Autodesk Fusion 360 part; units mm, degrees
note: some values were not read from the file. Set by a fixed rule: which sketch regions a step uses.
(part 2 of 2)
  spline S9 degree 5 poles (41.1532, -1.6486) (41.1603, -1.6542) (41.1746, -1.6654) (41.1961, -1.6821) (41.2247, -1.7041) (41.2607, -1.7314) (41.2967, -1.7583) (41.3329, -1.7849) (41.3691, -1.8112) (41.4054, -1.8372) (41.4419, -1.8628) (41.4784, -1.8881) (41.515, -1.9131) (41.5517, -1.9378) (41.5885, -1.9621) (41.6254, -1.9861) (41.6623, -2.0097) (41.6994, -2.033) (41.7365, -2.056) (41.7737, -2.0786) (41.811, -2.1009) (41.8483, -2.1229) (41.8857, -2.1445) (41.9232, -2.1657) (41.9608, -2.1866) (41.9984, -2.2071) (42.0361, -2.2273) (42.0738, -2.2471) (42.1116, -2.2666) (42.1495, -2.2857) (42.1874, -2.3044) (42.2254, -2.3227) (42.2634, -2.3407) (42.3014, -2.3583) (42.3395, -2.3755) (42.3777, -2.3923) (42.4158, -2.4088) (42.4541, -2.4248) (42.4923, -2.4405) (42.5306, -2.4558) (42.5689, -2.4706) (42.6072, -2.4851) (42.6456, -2.4991) (42.684, -2.5127) (42.7224, -2.5259) (42.7608, -2.5387) (42.7992, -2.551) (42.8377, -2.563) (42.8761, -2.5745) (42.9145, -2.5855) (42.953, -2.5961) (42.9914, -2.6063) (43.0299, -2.6159) (43.0683, -2.625) (43.1067, -2.6336) (43.145, -2.6417) (43.1834, -2.6494) (43.2217, -2.6566) (43.2601, -2.6634) (43.2983, -2.6697) (43.3366, -2.6753) (43.3747, -2.6802) (43.4128, -2.6844) (43.4508, -2.6877) (43.4888, -2.6904) (43.5266, -2.6925) (43.5644, -2.6943) (43.6022, -2.6956) (43.6398, -2.6965) (43.6773, -2.6964) (43.7146, -2.6948) (43.7442, -2.6918) (43.7662, -2.6883) (43.7808, -2.6855) (43.7881, -2.684) knots -1 -1 -1 -1 -1 -1 -0.98571429 -0.97142857 -0.95714286 -0.94285714 -0.92857143 -0.91428571 -0.9 -0.88571429 -0.87142857 -0.85714286 -0.84285714 -0.82857143 -0.81428571 -0.8 -0.78571429 -0.77142857 -0.75714286 -0.74285714 -0.72857143 -0.71428571 -0.7 -0.68571429 -0.67142857 -0.65714286 -0.64285714 -0.62857143 -0.61428571 -0.6 -0.58571429 -0.57142857 -0.55714286 -0.54285714 -0.52857143 -0.51428571 -0.5 -0.48571429 -0.47142857 -0.45714286 -0.44285714 -0.42857143 -0.41428571 -0.4 -0.38571429 -0.37142857 -0.35714286 -0.34285714 -0.32857143 -0.31428571 -0.3 -0.28571429 -0.27142857 -0.25714286 -0.24285714 -0.22857143 -0.21428571 -0.2 -0.18571429 -0.17142857 -0.15714286 -0.14285714 -0.12857143 -0.11428571 -0.1 -0.08571429 -0.07142857 -0.05714286 -0.04285714 -0.02857143 -0.01428571 0 0 0 0 0 0
  line L9 (43.7881, -2.684) -> (44.8114, -2.4656)
  arc A19 (45.9543, -3.0869) -> (44.8114, -2.4656) centre (45.0201, -3.4436) ccw
  arc A20 (45.9543, -3.0869) -> (46.0732, -3.3739) centre (51.1385, -1.1076) ccw
  arc A21 (45.7044, -4.6213) -> (46.0732, -3.3739) centre (45.1604, -3.7822) ccw
  line L10 (45.7044, -4.6213) -> (44.8264, -5.1905)
  spline S10 degree 5 poles (44.8264, -5.1905) (44.8201, -5.1946) (44.8078, -5.2029) (44.7898, -5.2161) (44.7668, -5.2349) (44.7393, -5.2601) (44.7127, -5.2865) (44.6866, -5.3138) (44.6609, -5.3414) (44.6354, -5.3694) (44.6102, -5.3977) (44.5852, -5.4264) (44.5607, -5.4557) (44.5367, -5.4855) (44.5132, -5.516) (44.4902, -5.547) (44.4675, -5.5785) (44.4452, -5.6104) (44.4232, -5.6426) (44.4015, -5.6751) (44.3801, -5.708) (44.3591, -5.7413) (44.3384, -5.7749) (44.318, -5.8088) (44.298, -5.8432) (44.2783, -5.8778) (44.2589, -5.9129) (44.2399, -5.9482) (44.2211, -5.9838) (44.2027, -6.0197) (44.1845, -6.0559) (44.1667, -6.0924) (44.1492, -6.1291) (44.132, -6.1662) (44.1151, -6.2035) (44.0985, -6.2411) (44.0823, -6.279) (44.0663, -6.3171) (44.0506, -6.3555) (44.0353, -6.3941) (44.0202, -6.433) (44.0054, -6.4721) (43.9909, -6.5114) (43.9768, -6.551) (43.9629, -6.5908) (43.9493, -6.6309) (43.9361, -6.6711) (43.9231, -6.7116) (43.9104, -6.7523) (43.898, -6.7932) (43.886, -6.8344) (43.8742, -6.8757) (43.8627, -6.9172) (43.8515, -6.9589) (43.8406, -7.0009) (43.83, -7.043) (43.8197, -7.0853) (43.8097, -7.1278) (43.8, -7.1705) (43.7906, -7.2133) (43.7815, -7.2564) (43.7726, -7.2996) (43.7641, -7.343) (43.7559, -7.3865) (43.748, -7.4302) (43.7403, -7.4741) (43.733, -7.5182) (43.726, -7.5624) (43.7192, -7.6068) (43.7128, -7.6513) (43.7066, -7.696) (43.702, -7.7318) (43.6986, -7.7588) (43.6964, -7.7768) (43.6953, -7.7858) knots 0 0 0 0 0 0 0.01428571 0.02857143 0.04285714 0.05714286 0.07142857 0.08571429 0.1 0.11428571 0.12857143 0.14285714 0.15714286 0.17142857 0.18571429 0.2 0.21428571 0.22857143 0.24285714 0.25714286 0.27142857 0.28571429 0.3 0.31428571 0.32857143 0.34285714 0.35714286 0.37142857 0.38571429 0.4 0.41428571 0.42857143 0.44285714 0.45714286 0.47142857 0.48571429 0.5 0.51428571 0.52857143 0.54285714 0.55714286 0.57142857 0.58571429 0.6 0.61428571 0.62857143 0.64285714 0.65714286 0.67142857 0.68571429 0.7 0.71428571 0.72857143 0.74285714 0.75714286 0.77142857 0.78571429 0.8 0.81428571 0.82857143 0.84285714 0.85714286 0.87142857 0.88571429 0.9 0.91428571 0.92857143 0.94285714 0.95714286 0.97142857 0.98571429 1 1 1 1 1 1
  arc A22 (43.6953, -7.7858) -> (44.4604, -8.5509) centre (51.1385, -1.1076) ccw
  spline S11 degree 5 poles (44.4604, -8.5509) (44.4694, -8.5498) (44.4874, -8.5476) (44.5144, -8.5442) (44.5502, -8.5396) (44.5949, -8.5334) (44.6394, -8.527) (44.6838, -8.5202) (44.728, -8.5132) (44.7721, -8.5058) (44.8159, -8.4982) (44.8597, -8.4903) (44.9032, -8.4821) (44.9466, -8.4735) (44.9898, -8.4647) (45.0329, -8.4556) (45.0757, -8.4462) (45.1184, -8.4365) (45.1609, -8.4265) (45.2032, -8.4162) (45.2453, -8.4056) (45.2873, -8.3947) (45.329, -8.3835) (45.3705, -8.372) (45.4118, -8.3602) (45.453, -8.3482) (45.4939, -8.3358) (45.5346, -8.3231) (45.575, -8.3101) (45.6153, -8.2969) (45.6554, -8.2833) (45.6952, -8.2694) (45.7347, -8.2552) (45.7741, -8.2408) (45.8132, -8.226) (45.8521, -8.2109) (45.8907, -8.1956) (45.9291, -8.1799) (45.9672, -8.1639) (46.0051, -8.1476) (46.0427, -8.1311) (46.08, -8.1142) (46.117, -8.097) (46.1538, -8.0795) (46.1903, -8.0616) (46.2265, -8.0435) (46.2624, -8.0251) (46.298, -8.0063) (46.3333, -7.9873) (46.3683, -7.9679) (46.403, -7.9482) (46.4374, -7.9282) (46.4713, -7.9078) (46.5049, -7.8871) (46.5382, -7.866) (46.5711, -7.8447) (46.6036, -7.823) (46.6358, -7.801) (46.6677, -7.7787) (46.6992, -7.756) (46.7302, -7.733) (46.7607, -7.7095) (46.7905, -7.6855) (46.8198, -7.661) (46.8485, -7.636) (46.8768, -7.6108) (46.9048, -7.5853) (46.9324, -7.5595) (46.9597, -7.5335) (46.9861, -7.5069) (47.0113, -7.4794) (47.0301, -7.4564) (47.0433, -7.4384) (47.0516, -7.426) (47.0556, -7.4198) knots -1 -1 -1 -1 -1 -1 -0.98571429 -0.97142857 -0.95714286 -0.94285714 -0.92857143 -0.91428571 -0.9 -0.88571429 -0.87142857 -0.85714286 -0.84285714 -0.82857143 -0.81428571 -0.8 -0.78571429 -0.77142857 -0.75714286 -0.74285714 -0.72857143 -0.71428571 -0.7 -0.68571429 -0.67142857 -0.65714286 -0.64285714 -0.62857143 -0.61428571 -0.6 -0.58571429 -0.57142857 -0.55714286 -0.54285714 -0.52857143 -0.51428571 -0.5 -0.48571429 -0.47142857 -0.45714286 -0.44285714 -0.42857143 -0.41428571 -0.4 -0.38571429 -0.37142857 -0.35714286 -0.34285714 -0.32857143 -0.31428571 -0.3 -0.28571429 -0.27142857 -0.25714286 -0.24285714 -0.22857143 -0.21428571 -0.2 -0.18571429 -0.17142857 -0.15714286 -0.14285714 -0.12857143 -0.11428571 -0.1 -0.08571429 -0.07142857 -0.05714286 -0.04285714 -0.02857143 -0.01428571 0 0 0 0 0 0
  line L11 (47.0556, -7.4198) -> (47.6248, -6.5418)
  arc A23 (48.8723, -6.173) -> (47.6248, -6.5418) centre (48.4639, -7.0858) ccw
  arc A24 (48.8723, -6.173) -> (49.1593, -6.2918) centre (51.1385, -1.1076) ccw
  arc A25 (49.7806, -7.4347) -> (49.1593, -6.2918) centre (48.8026, -7.2261) ccw
  line L12 (49.7806, -7.4347) -> (49.5622, -8.4581)
  spline S12 degree 5 poles (49.5622, -8.4581) (49.5607, -8.4653) (49.5578, -8.48) (49.5544, -8.502) (49.5514, -8.5316) (49.5498, -8.5688) (49.5497, -8.6063) (49.5505, -8.644) (49.5519, -8.6817) (49.5537, -8.7196) (49.5558, -8.7574) (49.5585, -8.7954) (49.5618, -8.8334) (49.566, -8.8715) (49.5709, -8.9096) (49.5765, -8.9479) (49.5828, -8.9861) (49.5895, -9.0244) (49.5968, -9.0628) (49.6045, -9.1011) (49.6126, -9.1395) (49.6212, -9.1779) (49.6303, -9.2163) (49.6399, -9.2548) (49.65, -9.2932) (49.6606, -9.3316) (49.6717, -9.3701) (49.6832, -9.4085) (49.6951, -9.447) (49.7075, -9.4854) (49.7203, -9.5238) (49.7335, -9.5622) (49.7471, -9.6006) (49.7611, -9.6389) (49.7756, -9.6773) (49.7904, -9.7156) (49.8057, -9.7539) (49.8214, -9.7921) (49.8374, -9.8303) (49.8539, -9.8685) (49.8707, -9.9067) (49.8879, -9.9448) (49.9055, -9.9828) (49.9235, -10.0208) (49.9418, -10.0588) (49.9605, -10.0967) (49.9796, -10.1346) (49.9991, -10.1724) (50.0189, -10.2101) (50.0391, -10.2478) (50.0596, -10.2854) (50.0805, -10.323) (50.1017, -10.3604) (50.1233, -10.3979) (50.1453, -10.4352) (50.1675, -10.4725) (50.1902, -10.5097) (50.2131, -10.5468) (50.2365, -10.5838) (50.2601, -10.6208) (50.2841, -10.6577) (50.3084, -10.6945) (50.3331, -10.7312) (50.3581, -10.7678) (50.3834, -10.8043) (50.409, -10.8408) (50.435, -10.8771) (50.4613, -10.9133) (50.4879, -10.9495) (50.5148, -10.9855) (50.542, -11.0214) (50.5641, -11.0501) (50.5808, -11.0716) (50.5919, -11.0859) (50.5976, -11.093) knots 0 0 0 0 0 0 0.01428571 0.02857143 0.04285714 0.05714286 0.07142857 0.08571429 0.1 0.11428571 0.12857143 0.14285714 0.15714286 0.17142857 0.18571429 0.2 0.21428571 0.22857143 0.24285714 0.25714286 0.27142857 0.28571429 0.3 0.31428571 0.32857143 0.34285714 0.35714286 0.37142857 0.38571429 0.4 0.41428571 0.42857143 0.44285714 0.45714286 0.47142857 0.48571429 0.5 0.51428571 0.52857143 0.54285714 0.55714286 0.57142857 0.58571429 0.6 0.61428571 0.62857143 0.64285714 0.65714286 0.67142857 0.68571429 0.7 0.71428571 0.72857143 0.74285714 0.75714286 0.77142857 0.78571429 0.8 0.81428571 0.82857143 0.84285714 0.85714286 0.87142857 0.88571429 0.9 0.91428571 0.92857143 0.94285714 0.95714286 0.97142857 0.98571429 1 1 1 1 1 1
  arc A26 (50.5976, -11.093) -> (51.6795, -11.093) centre (51.1385, -1.1076) ccw
  spline S13 degree 5 poles (51.6795, -11.093) (51.6852, -11.0859) (51.6963, -11.0716) (51.713, -11.0501) (51.7351, -11.0214) (51.7623, -10.9855) (51.7892, -10.9495) (51.8158, -10.9133) (51.8421, -10.8771) (51.8681, -10.8408) (51.8937, -10.8043) (51.919, -10.7678) (51.944, -10.7312) (51.9687, -10.6945) (51.993, -10.6577) (52.017, -10.6208) (52.0406, -10.5838) (52.064, -10.5468) (52.0869, -10.5097) (52.1096, -10.4725) (52.1318, -10.4352) (52.1538, -10.3979) (52.1754, -10.3604) (52.1966, -10.323) (52.2175, -10.2854) (52.238, -10.2478) (52.2582, -10.2101) (52.278, -10.1724) (52.2975, -10.1346) (52.3166, -10.0967) (52.3353, -10.0588) (52.3536, -10.0208) (52.3716, -9.9828) (52.3892, -9.9448) (52.4064, -9.9067) (52.4232, -9.8685) (52.4397, -9.8303) (52.4557, -9.7921) (52.4714, -9.7539) (52.4867, -9.7156) (52.5015, -9.6773) (52.516, -9.6389) (52.53, -9.6006) (52.5436, -9.5622) (52.5568, -9.5238) (52.5696, -9.4854) (52.582, -9.447) (52.5939, -9.4085) (52.6054, -9.3701) (52.6165, -9.3316) (52.6271, -9.2932) (52.6372, -9.2548) (52.6468, -9.2163) (52.6559, -9.1779) (52.6645, -9.1395) (52.6726, -9.1011) (52.6803, -9.0628) (52.6875, -9.0244) (52.6943, -8.9861) (52.7006, -8.9479) (52.7062, -8.9096) (52.7111, -8.8715) (52.7153, -8.8334) (52.7186, -8.7954) (52.7213, -8.7574) (52.7234, -8.7196) (52.7252, -8.6817) (52.7266, -8.644) (52.7274, -8.6063) (52.7273, -8.5688) (52.7257, -8.5316) (52.7227, -8.502) (52.7193, -8.48) (52.7164, -8.4653) (52.7149, -8.4581) knots -1 -1 -1 -1 -1 -1 -0.98571429 -0.97142857 -0.95714286 -0.94285714 -0.92857143 -0.91428571 -0.9 -0.88571429 -0.87142857 -0.85714286 -0.84285714 -0.82857143 -0.81428571 -0.8 -0.78571429 -0.77142857 -0.75714286 -0.74285714 -0.72857143 -0.71428571 -0.7 -0.68571429 -0.67142857 -0.65714286 -0.64285714 -0.62857143 -0.61428571 -0.6 -0.58571429 -0.57142857 -0.55714286 -0.54285714 -0.52857143 -0.51428571 -0.5 -0.48571429 -0.47142857 -0.45714286 -0.44285714 -0.42857143 -0.41428571 -0.4 -0.38571429 -0.37142857 -0.35714286 -0.34285714 -0.32857143 -0.31428571 -0.3 -0.28571429 -0.27142857 -0.25714286 -0.24285714 -0.22857143 -0.21428571 -0.2 -0.18571429 -0.17142857 -0.15714286 -0.14285714 -0.12857143 -0.11428571 -0.1 -0.08571429 -0.07142857 -0.05714286 -0.04285714 -0.02857143 -0.01428571 0 0 0 0 0 0
  line L13 (52.7149, -8.4581) -> (52.4965, -7.4347)
  arc A27 (53.1178, -6.2918) -> (52.4965, -7.4347) centre (53.4745, -7.2261) ccw
  arc A28 (53.1178, -6.2918) -> (53.4048, -6.173) centre (51.1385, -1.1076) ccw
  arc A29 (54.6523, -6.5418) -> (53.4048, -6.173) centre (53.8132, -7.0858) ccw
  line L14 (54.6523, -6.5418) -> (55.2214, -7.4198)
  spline S14 degree 5 poles (55.2214, -7.4198) (55.2255, -7.426) (55.2338, -7.4384) (55.247, -7.4564) (55.2658, -7.4794) (55.291, -7.5069) (55.3174, -7.5335) (55.3447, -7.5595) (55.3723, -7.5853) (55.4003, -7.6108) (55.4286, -7.636) (55.4573, -7.661) (55.4866, -7.6855) (55.5164, -7.7095) (55.5469, -7.733) (55.5779, -7.756) (55.6094, -7.7787) (55.6413, -7.801) (55.6735, -7.823) (55.706, -7.8447) (55.7389, -7.866) (55.7722, -7.8871) (55.8058, -7.9078) (55.8397, -7.9282) (55.8741, -7.9482) (55.9088, -7.9679) (55.9438, -7.9873) (55.9791, -8.0063) (56.0147, -8.0251) (56.0506, -8.0435) (56.0868, -8.0616) (56.1233, -8.0795) (56.16, -8.097) (56.1971, -8.1142) (56.2344, -8.1311) (56.272, -8.1476) (56.3099, -8.1639) (56.348, -8.1799) (56.3864, -8.1956) (56.425, -8.2109) (56.4639, -8.226) (56.503, -8.2408) (56.5424, -8.2552) (56.5819, -8.2694) (56.6217, -8.2833) (56.6618, -8.2969) (56.7021, -8.3101) (56.7425, -8.3231) (56.7832, -8.3358) (56.8241, -8.3482) (56.8653, -8.3602) (56.9066, -8.372) (56.9481, -8.3835) (56.9898, -8.3947) (57.0318, -8.4056) (57.0739, -8.4162) (57.1162, -8.4265) (57.1587, -8.4365) (57.2014, -8.4462) (57.2442, -8.4556) (57.2873, -8.4647) (57.3305, -8.4735) (57.3739, -8.4821) (57.4174, -8.4903) (57.4612, -8.4982) (57.505, -8.5058) (57.5491, -8.5132) (57.5933, -8.5202) (57.6377, -8.527) (57.6822, -8.5334) (57.7269, -8.5396) (57.7627, -8.5442) (57.7897, -8.5476) (57.8077, -8.5498) (57.8167, -8.5509) knots 0 0 0 0 0 0 0.01428571 0.02857143 0.04285714 0.05714286 0.07142857 0.08571429 0.1 0.11428571 0.12857143 0.14285714 0.15714286 0.17142857 0.18571429 0.2 0.21428571 0.22857143 0.24285714 0.25714286 0.27142857 0.28571429 0.3 0.31428571 0.32857143 0.34285714 0.35714286 0.37142857 0.38571429 0.4 0.41428571 0.42857143 0.44285714 0.45714286 0.47142857 0.48571429 0.5 0.51428571 0.52857143 0.54285714 0.55714286 0.57142857 0.58571429 0.6 0.61428571 0.62857143 0.64285714 0.65714286 0.67142857 0.68571429 0.7 0.71428571 0.72857143 0.74285714 0.75714286 0.77142857 0.78571429 0.8 0.81428571 0.82857143 0.84285714 0.85714286 0.87142857 0.88571429 0.9 0.91428571 0.92857143 0.94285714 0.95714286 0.97142857 0.98571429 1 1 1 1 1 1
  arc A30 (57.8167, -8.5509) -> (58.5818, -7.7858) centre (51.1385, -1.1076) ccw
  spline S15 degree 5 poles (58.5818, -7.7858) (58.5807, -7.7768) (58.5785, -7.7588) (58.5751, -7.7318) (58.5705, -7.696) (58.5643, -7.6513) (58.5579, -7.6068) (58.5511, -7.5624) (58.5441, -7.5182) (58.5368, -7.4741) (58.5291, -7.4302) (58.5212, -7.3865) (58.513, -7.343) (58.5045, -7.2996) (58.4956, -7.2564) (58.4865, -7.2133) (58.4771, -7.1705) (58.4674, -7.1278) (58.4574, -7.0853) (58.4471, -7.043) (58.4365, -7.0009) (58.4256, -6.9589) (58.4144, -6.9172) (58.4029, -6.8757) (58.3911, -6.8344) (58.3791, -6.7932) (58.3667, -6.7523) (58.354, -6.7116) (58.341, -6.6711) (58.3278, -6.6309) (58.3142, -6.5908) (58.3003, -6.551) (58.2862, -6.5114) (58.2717, -6.4721) (58.2569, -6.433) (58.2418, -6.3941) (58.2265, -6.3555) (58.2108, -6.3171) (58.1948, -6.279) (58.1786, -6.2411) (58.162, -6.2035) (58.1451, -6.1662) (58.1279, -6.1291) (58.1104, -6.0924) (58.0926, -6.0559) (58.0744, -6.0197) (58.056, -5.9838) (58.0372, -5.9482) (58.0182, -5.9129) (57.9988, -5.8778) (57.9791, -5.8432) (57.9591, -5.8088) (57.9387, -5.7749) (57.918, -5.7413) (57.897, -5.708) (57.8756, -5.6751) (57.8539, -5.6426) (57.8319, -5.6104) (57.8096, -5.5785) (57.7869, -5.547) (57.7639, -5.516) (57.7404, -5.4855) (57.7164, -5.4557) (57.6919, -5.4264) (57.6669, -5.3977) (57.6417, -5.3694) (57.6162, -5.3414) (57.5905, -5.3138) (57.5644, -5.2865) (57.5378, -5.2601) (57.5103, -5.2349) (57.4873, -5.2161) (57.4693, -5.2029) (57.457, -5.1946) (57.4507, -5.1905) knots -1 -1 -1 -1 -1 -1 -0.98571429 -0.97142857 -0.95714286 -0.94285714 -0.92857143 -0.91428571 -0.9 -0.88571429 -0.87142857 -0.85714286 -0.84285714 -0.82857143 -0.81428571 -0.8 -0.78571429 -0.77142857 -0.75714286 -0.74285714 -0.72857143 -0.71428571 -0.7 -0.68571429 -0.67142857 -0.65714286 -0.64285714 -0.62857143 -0.61428571 -0.6 -0.58571429 -0.57142857 -0.55714286 -0.54285714 -0.52857143 -0.51428571 -0.5 -0.48571429 -0.47142857 -0.45714286 -0.44285714 -0.42857143 -0.41428571 -0.4 -0.38571429 -0.37142857 -0.35714286 -0.34285714 -0.32857143 -0.31428571 -0.3 -0.28571429 -0.27142857 -0.25714286 -0.24285714 -0.22857143 -0.21428571 -0.2 -0.18571429 -0.17142857 -0.15714286 -0.14285714 -0.12857143 -0.11428571 -0.1 -0.08571429 -0.07142857 -0.05714286 -0.04285714 -0.02857143 -0.01428571 0 0 0 0 0 0
  line L15 (57.4507, -5.1905) -> (56.5727, -4.6213)
  arc A31 (56.2039, -3.3739) -> (56.5727, -4.6213) centre (57.1167, -3.7822) ccw
  circle A32 centre (51.1385, -1.1076) radius 0.5
  line L16 (51.1385, -1.1076) -> (52.7158, 0.3015)
  circle A33 centre (52.7158, 0.3015) radius 0.5
  point P0 (51.1385, -1.1076)
  dimension "d255" = 2.115
  dimension "d256" = 1
  constraint coincident P0 A0.centre
  constraint coincident L16.end A33.centre
  measures "d255" distance of P0 L16.end
  measures "d256" diameter of A33
hole "Hole1" at (1.5771, 1.418, 0.5) direction (0, 0, -1) diameter 1 depth 2 tip angle 118 bodies 41 in component "Spur Gear (8 teeth)"
extrude "Extrude9" [suppressed]
component "Component" placed x (0.827972, 0, 0.560769) y (0, 1, 0) z (-0.560769, 0, 0.827972) at (9.8094, 0, -23.0724)
component "Component'" placed x (-0.964215, 0, 0.265122) y (0, 1, 0) z (-0.265122, 0, -0.964215) at (78.5301, 0, -2.3257)
component "Component''" placed x (0.93362, 0, -0.358265) y (0, 1, 0) z (0.358265, 0, 0.93362) at (-5.5018, 0, -4.2163)
component "Component'''" placed x (1, 0, 0) y (0, 1, 0) z (0, 0, 1) at (-14.129, 0, 11.489)
component "Component''''" placed x (1, 0, 0) y (0, 1, 0) z (0, 0, 1) at (20.8, 0, 4.5)
component "Component'''''" placed x (1, 0, 0) y (0, 1, 0) z (0, 0, 1) at (42.51, 0, 4.452)
component "Component''''''" placed x (1, 0, 0) y (0, 1, 0) z (0, 0, 1) at (39.422, 0, 4.137)
component "Component'''''''" placed x (0.784272, 0, -0.620417) y (0, 1, 0) z (0.620417, 0, 0.784272) at (-14.037, -0.5, 3.1654)
component "Component''''''''" placed x (0.993496, 0, -0.11387) y (0, 1, 0) z (0.11387, 0, 0.993496) at (-1.4667, -1, 7.9441)
component "Component'''''''''" placed x (0.999998, 0, 0.001926) y (0, 1, 0) z (-0.001926, 0, 0.999998) at (0.0282, -1, 43.3562)
component "Component''''''''''" placed x (0.990388, 0, 0.138316) y (0, 1, 0) z (-0.138316, 0, 0.990388) at (6.7019, 0.5, 51.2293)
component "Component'''''''''''" placed x (-0.501631, 0, 0.865082) y (0, 1, 0) z (-0.865082, 0, -0.501631) at (-15.1691, -0.5, -17.1877)
component "Component''''''''''''" placed x (-0.701941, 0, 0.712235) y (0, 1, 0) z (-0.712235, 0, -0.701941) at (-18.5612, -0.5, -6.5985)
component "Component'''''''''''''" placed x (0.999998, 0, 0.001926) y (0, 1, 0) z (-0.001926, 0, 0.999998) at (12.0419, -0.5, 36.252)
component "Component''''''''''''''" placed x (0.678456, 0, -0.734641) y (0, 1, 0) z (0.734641, 0, 0.678456) at (27.2088, -2, -8.0294)
component "Component'''''''''''''''" placed x (0.674831, 0, 0.737972) y (0, 1, 0) z (-0.737972, 0, 0.674831) at (16.9413, -1, 39.8056)
component "Component''''''''''''''''" placed x (0.489595, 0, -0.87195) y (0, -1, 0) z (-0.87195, 0, -0.489595) at (-10.5813, -2, -9.7893)
component "Component'''''''''''''''''" placed x (0.489595, 0, -0.87195) y (0, -1, 0) z (-0.87195, 0, -0.489595) at (-5.3992, -2.5, -0.5719)
component "Component''''''''''''''''''" placed x (0.485497, 0, 0.874239) y (0, -1, 0) z (0.874239, 0, -0.485497) at (35.3206, -1.5, 17.8648)
component "Component'''''''''''''''''''" placed x (0.485497, 0, 0.874239) y (0, 1, 0) z (-0.874239, 0, 0.485497) at (-3.4139, -1.5, 32.5124)
component "Spur Gear (8 teeth)" placed x (-0.990388, 0, -0.138316) y (0.138316, 0, -0.990388) z (0, -1, 0) at (20.8, 0, 4.5)
